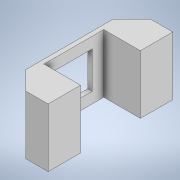
# Autodesk Inventor part: latticeChamberHolderv1
Saved by Autodesk Inventor 2020 (Build 240168000, 168)
## iProperties
Created: 2022-09-27
Part Number: latticeChamberHolderv1
Material: Generic
Document SubType Name: Modeling
Designer: iss
Density: 1 g/cm^3
Appearance: Default
Author: iss
Autodesk Inventor part; units mm, degrees
ref_plane "YZ Plane" through (0, 0, 0) normal (1, 0, 0) x (0, 1, 0)
ref_plane "XZ Plane" through (0, 0, 0) normal (0, 1, 0) x (-1, 0, 0)
ref_plane "XY Plane" through (0, 0, 0) normal (0, 0, 1) x (1, 0, 0)
sketch "Sketch1" plane through (0, 0, 0) normal (0, 1, 0) x (-1, 0, 0)
  line L0 (0, 0) -> (0, -11.468)
  line L1 (0, -11.468) -> (7.909, -11.468)
  line L2 (14.366, -5.011) -> (14.366, 10)
  line L3 (12.5, 10) -> (0, 10)
  line L4 (14.366, -5.011) -> (7.909, -11.468)
  line L5 (0, 0) -> (12.5, 0)
  line L6 (12.5, 0) -> (12.5, 10)
  line L7 (0, 20) -> (0, 31.468)
  line L8 (0, 31.468) -> (7.909, 31.468)
  line L9 (14.366, 25.011) -> (14.366, 10)
  line L10 (14.366, 25.011) -> (7.909, 31.468)
  line L11 (0, 20) -> (12.5, 20)
  line L12 (12.5, 20) -> (12.5, 10)
  line L13 (0.2, -11.268) -> (0.2, -0.2)
  line L14 (0.2, -0.2) -> (12.7, -0.2)
  line L15 (12.7, -0.2) -> (12.7, 10)
  line L16 (12.7, 10) -> (12.7, 20.2)
  line L17 (12.7, 20.2) -> (0.2, 20.2)
  line L18 (0.2, 20.2) -> (0.2, 31.268)
  line L19 (0.2, 31.268) -> (7.8262, 31.268)
  line L20 (7.8262, 31.268) -> (14.166, 24.9282)
  line L21 (14.166, 24.9282) -> (14.166, 10)
  line L22 (14.166, 10) -> (14.166, -4.9282)
  line L23 (14.166, -4.9282) -> (7.8262, -11.268)
  line L24 (7.8262, -11.268) -> (0.2, -11.268)
  point P0 (14.366, -11.468)
  point P1 (14.366, 31.468)
  dimension "d0" = 11.468
  dimension "d1" = 14.366
  dimension "d2" = 21.468
  dimension "d3" = 6.457
  dimension "d4" = 6.457
  dimension "d5" = 12.5
  dimension "d8" = 0.2
  constraints: 50 end point, 6 symmetric about line, 4 point on line, 2 horizontal, 2 perpendicular, 2 vertical, 11 other
  measures "d0" distance of L0.start L0.end
  measures "d1" distance of L0.end point (14.366, -11.468)
  measures "d2" distance of point (14.366, -11.468) L2.end
  measures "d3" distance of L2.start point (14.366, -11.468)
  measures "d4" distance of L1.end point (14.366, -11.468)
  measures "d5" distance of L0.start L5.end
  measures "d8" distance between parallel lines of L0 L13
extrude "Extrusion1" add sketch "Sketch1" along normal blind 20 contours L13 L14 L15 L16 L17 L18 L19 L20 L21 L22 L23 L24
sketch "Sketch2" plane through (-14.166, 0, -4.9282) normal (-1, 0, 0) x (0, 0, 1)
  line L0 (0, 0) -> (29.8563, 0) projected
  line L1 (29.8563, 0) -> (29.8563, 20) projected
  line L2 (0, 20) -> (29.8563, 20) projected
  line L3 (0, 0) -> (0, 20) projected
  line L4 (0, 20) -> (29.8563, 20) projected
  line L5 (14.9282, 20) -> (14.9282, 0)
  line L6 (0, 0) -> (29.8563, 0) projected
  line L7 (29.8563, 0) -> (29.8563, 20) projected
  line L8 (29.8563, 10) -> (0, 10)
  line L9 (0, 0) -> (0, 20) projected
  line L10 (8.6782, 16.25) -> (21.1782, 16.25)
  line L11 (21.1782, 16.25) -> (21.1782, 3.75)
  line L12 (21.1782, 3.75) -> (8.6782, 3.75)
  line L13 (8.6782, 3.75) -> (8.6782, 16.25)
  point P0 (4.9282, 0)
  dimension "d8" = 0.2
  dimension "d9" = 12.5
  dimension "d10" = 12.5
  dimension "d11" = 6.25
  dimension "d12" = 6.25
  constraints: 12 end point, 4 midpoint, 2 parallel, 1 horizontal, 1 perpendicular
  measures "d9" distance of L11.end L12.end
  measures "d10" distance of L10.end L11.end
  measures "d11" distance between parallel lines of L5 L11
  measures "d12" distance between parallel lines of L8 L10
extrude "Extrusion2" cut sketch "Sketch2" against normal blind 20 contours L12 L13 L8 L5 | L5 L8 L11 L12 | L13 L10 L5 L8 | L5 L10 L11 L8
equation "\"d4\" = d3"
body "Solid1"
